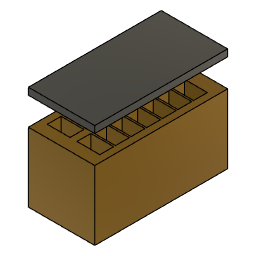
Sertraline 50or100 v0 (Autodesk Fusion 360 design; units mm, degrees)
Autodesk Fusion 360 part; units mm, degrees
note: some values were not read from the file. Chosen so that the rebuilt part matches the saved one: which face or edge a step refers to; a direction.
sketch "Sketch1" plane through (0, 0, 0) normal (0, 0, 1) x (1, 0, 0)
  line L0 (32.9923, 14.7897) -> (80.9923, 14.7897)
  line L1 (80.9923, 14.7897) -> (80.9923, 110.7897)
  line L2 (80.9923, 110.7897) -> (32.9923, 110.7897)
  line L3 (32.9923, 110.7897) -> (32.9923, 14.7897)
  line L4 (56.9923, 110.7897) -> (56.9923, 14.7897)
  line L5 (56.9923, 110.7897) -> (56.9923, 101.7897)
  line L6 (56.9923, 14.7897) -> (56.9923, 22.7897)
  line L7 (56.9923, 22.7897) -> (56.9923, 34.0754)
  line L8 (56.9923, 34.0754) -> (56.9923, 45.3611)
  line L9 (56.9923, 45.3611) -> (56.9923, 56.6468)
  line L10 (56.9923, 56.6468) -> (56.9923, 67.9325)
  line L11 (56.9923, 67.9325) -> (56.9923, 79.2182)
  line L12 (56.9923, 79.2182) -> (56.9923, 90.5039)
  line L13 (56.9923, 90.5039) -> (56.9923, 101.7897)
  line L14 (56.9923, 101.7897) -> (56.9923, 101.1468)
  line L15 (56.9923, 90.5039) -> (56.9923, 91.1468)
  line L16 (56.9923, 90.5039) -> (56.9923, 89.8611)
  line L17 (56.9923, 79.2182) -> (56.9923, 79.8611)
  line L18 (56.9923, 79.2182) -> (56.9923, 78.5754)
  line L19 (56.9923, 67.9325) -> (56.9923, 68.5754)
  line L20 (56.9923, 67.9325) -> (56.9923, 67.2897)
  line L21 (56.9923, 56.6468) -> (56.9923, 57.2897)
  line L22 (56.9923, 56.6468) -> (56.9923, 56.0039)
  line L23 (56.9923, 45.3611) -> (56.9923, 46.0039)
  line L24 (56.9923, 45.3611) -> (56.9923, 44.7182)
  line L25 (56.9923, 34.0754) -> (56.9923, 34.7182)
  line L26 (56.9923, 34.0754) -> (56.9923, 33.4325)
  line L27 (56.9923, 22.7897) -> (56.9923, 23.4325)
  line L28 (32.9923, 101.1468) -> (80.9923, 101.1468)
  line L29 (80.9923, 91.1468) -> (32.9923, 91.1468)
  line L30 (80.9923, 89.8611) -> (32.9923, 89.8611)
  line L31 (80.9923, 79.8611) -> (32.9923, 79.8611)
  line L32 (80.9923, 78.5754) -> (32.9923, 78.5754)
  line L33 (80.9923, 68.5754) -> (32.9923, 68.5754)
  line L34 (80.9923, 67.2897) -> (32.9923, 67.2897)
  line L35 (80.9923, 57.2897) -> (32.9923, 57.2897)
  line L36 (80.9923, 56.0039) -> (32.9923, 56.0039)
  line L37 (80.9923, 46.0039) -> (32.9923, 46.0039)
  line L38 (80.9923, 44.7182) -> (32.9923, 44.7182)
  line L39 (80.9923, 34.7182) -> (32.9923, 34.7182)
  line L40 (80.9923, 33.4325) -> (32.9923, 33.4325)
  line L41 (80.9923, 23.4325) -> (32.9923, 23.4325)
  dimension "d1" = 48
  dimension "d2" = 96
  dimension "d3" = 9
  dimension "d4" = 8
  dimension "d5" = 11.2857
  dimension "d6" = 11.2857
  dimension "d7" = 11.2857
  dimension "d8" = 11.2857
  dimension "d9" = 11.2857
  dimension "d10" = 11.2857
  dimension "d11" = 11.2857
  dimension "d13" = 0.6429
  dimension "d14" = 0.6429
  dimension "d15" = 0.6429
  dimension "d16" = 0.6429
  dimension "d17" = 0.6429
  dimension "d18" = 0.6429
  dimension "d19" = 0.6429
  dimension "d20" = 0.6429
  dimension "d21" = 0.6429
  dimension "d22" = 0.6429
  dimension "d23" = 0.6429
  dimension "d24" = 0.6429
  dimension "d25" = 0.6429
  dimension "d26" = 0.6429
  constraint horizontal L0
  constraint vertical L1
  constraint horizontal L2
  constraint vertical L3
  constraint midpoint L2 L4.start
  constraint midpoint L0 L4.end
  constraint perpendicular L2 L5
  constraint perpendicular L0 L6
  constraint parallel L4 L7
  constraint parallel L4 L8
  constraint parallel L4 L9
  constraint parallel L4 L10
  constraint coincident L4 L11.end
  constraint coincident L4 L12.end
  constraint parallel L4 L13
  constraint vertical L14
  constraint vertical L15
  constraint parallel L4 L16
  constraint vertical L17
  constraint vertical L18
  constraint vertical L19
  constraint vertical L20
  constraint vertical L21
  constraint vertical L22
  constraint vertical L23
  constraint parallel L4 L24
  constraint parallel L8 L25
  constraint parallel L4 L26
  constraint parallel L4 L27
  constraint coincident L3 L28.start
  constraint coincident L1 L28.end
  constraint perpendicular L1 L28
  constraint coincident L1 L29.start
  constraint coincident L3 L29.end
  constraint perpendicular L3 L29
  constraint coincident L1 L30.start
  constraint coincident L3 L30.end
  constraint perpendicular L3 L30
  constraint coincident L1 L31.start
  constraint coincident L3 L31.end
  constraint perpendicular L3 L31
  constraint coincident L1 L32.start
  constraint coincident L3 L32.end
  constraint perpendicular L3 L32
  constraint coincident L1 L33.start
  constraint coincident L3 L33.end
  constraint perpendicular L3 L33
  constraint coincident L1 L34.start
  constraint coincident L3 L34.end
  constraint perpendicular L3 L34
  constraint coincident L3 L35.end
  constraint perpendicular L3 L35
  constraint coincident L1 L36.start
  constraint coincident L3 L36.end
  constraint perpendicular L3 L36
  constraint coincident L1 L37.start
  constraint coincident L3 L37.end
  constraint perpendicular L3 L37
  constraint coincident L3 L38.end
  constraint perpendicular L3 L38
  constraint coincident L1 L39.start
  constraint coincident L3 L39.end
  constraint perpendicular L3 L39
  constraint coincident L1 L40.start
  constraint coincident L3 L40.end
  constraint perpendicular L3 L40
  constraint coincident L1 L41.start
  constraint coincident L3 L41.end
  constraint perpendicular L3 L41
  measures "d1" distance of L0.start L0.end
  measures "d2" distance of L0.start L2.end
  measures "d3" distance of L4.start L5.end
  measures "d4" distance of L4.end L6.end
  measures "d5" distance of L6.end L7.end
  measures "d6" distance of L7.end L8.end
  measures "d7" distance of L8.end L9.end
  measures "d8" distance of L9.end L10.end
  measures "d9" distance of L10.end L11.end
  measures "d10" distance of L11.end L12.end
  measures "d11" distance of L12.end L5.end
  measures "d13" distance of L5.end L14.end
  measures "d14" distance of L12.end L15.end
  measures "d15" distance of L12.end L16.end
  measures "d16" distance of L11.end L17.end
  measures "d17" distance of L11.end L18.end
  measures "d18" distance of L10.end L19.end
  measures "d19" distance of L10.end L20.end
  measures "d20" distance of L9.end L21.end
  measures "d21" distance of L9.end L22.end
  measures "d22" distance of L8.end L23.end
  measures "d23" distance of L8.end L24.end
  measures "d24" distance of L7.end L25.end
  measures "d25" distance of L7.end L26.end
  measures "d26" distance of L6.end L27.end
extrude "Extrude1" add sketch "Sketch1" along normal blind 5 contours L0 L3 L4 L6 L7 L27 L41 | L0 L1 L4 L6 L7 L27 L41 | L3 L4 L7 L40 L41 | L1 L4 L7 L40 L41 | L3 L4 L8 L38 L39 | L1 L4 L8 L38 L39 | L3 L4 L9 L36 L37 | L1 L4 L9 L36 L37 | L3 L4 L10 L34 L35 | L1 L4 L10 L34 L35 | L3 L4 L11 L32 L33 | L1 L4 L11 L32 L33 | L3 L4 L12 L30 L31 | L1 L4 L12 L30 L31 | L3 L4 L13 L28 L29 | L2 L3 L4 L5 L13 L14 L28 | L1 L4 L13 L28 L29 | L1 L2 L4 L5 L13 L14 L28 makes body 1 at (48.9923, 49.3373, 0) makes body 2 at (64.9923, 97.6944, 0) makes body 3 at (48.9923, 60.623, 0) makes body 4 at (48.9923, 38.0516, 0) makes body 5 at (48.9923, 83.1944, 0) makes body 6 at (48.9923, 71.9087, 0) makes body 7 at (64.9923, 21.0039, 0)
sketch "Sketch2" plane through (0, 0, 5) normal (0, 0, 1) x (-1, 0, 0)
  line L0 (-80.9923, -110.7897) -> (-32.9923, -110.7897)
  line L1 (-32.9923, -110.7897) -> (-32.9923, -91.1468)
  line L2 (-32.9923, -91.1468) -> (-80.9923, -91.1468)
  line L3 (-80.9923, -91.1468) -> (-80.9923, -110.7897)
  line L4 (-32.9923, -110.7897) -> (-80.9923, -110.7897)
  line L5 (-80.9923, -110.7897) -> (-80.9923, -14.7897)
  line L6 (-80.9923, -14.7897) -> (-32.9923, -14.7897)
  line L7 (-32.9923, -14.7897) -> (-32.9923, -110.7897)
  point P0 (-80.9923, -14.7897)
  constraint horizontal L4
  constraint vertical L5
  constraint horizontal L6
  constraint vertical L7
  constraint coincident P0 L5.end
  constraint coincident L0.end L1.start
extrude "Extrude2" add sketch "Sketch2" along normal blind 5 bodies 1 2 3 4 5 6 7
sketch "Sketch3" plane through (0, 0, 0) normal (0, 0, -1) x (1, 0, 0)
  line L0 (32.9923, -67.2897) -> (80.9923, -67.2897)
  line L1 (80.9923, -67.2897) -> (80.9923, -57.2897)
  line L2 (80.9923, -57.2897) -> (32.9923, -57.2897)
  line L3 (32.9923, -57.2897) -> (32.9923, -67.2897)
  line L4 (56.9923, -62.2897) -> (56.9923, -10.4261)
  line L5 (56.9923, -10.4261) -> (54.4923, -10.4261)
  line L6 (54.4923, -10.4261) -> (59.4923, -10.4261)
  line L7 (59.4923, -10.4261) -> (59.4923, -116.1446)
  line L8 (59.4923, -116.1446) -> (54.4923, -116.1446)
  line L9 (54.4923, -116.1446) -> (54.4923, -10.4261)
  dimension "d32" = 2.5
  dimension "d33" = 5
  constraint perpendicular L2 L4
  constraint perpendicular L4 L5
  constraint horizontal L6
  constraint vertical L7
  constraint horizontal L8
  constraint vertical L9
  measures "d32" distance of L4.end L5.end
  measures "d33" distance of L5.end L6.end
extrude "Extrude3" cut sketch "Sketch3" against normal blind 5 contours L0 L2 L7 L9 | L0 L7 L8 L9 | L2 L4 L5 L6 L9 | L2 L4 L6 L7 bodies 1
sketch "Sketch4" plane through (0, 0, 0) normal (0, 0, 1) x (1, 0, 0)
extrude "Extrude4" cut sketch "Sketch1" along normal blind 5 contours L2 L3 L4 L5 L13 L14 L28 | L1 L2 L4 L5 L13 L14 L28 bodies 1
extrude "Extrude5" cut sketch "Sketch1" along normal blind 5 contours L0 L3 L4 L6 L7 L27 L41 | L0 L1 L4 L6 L7 L27 L41 bodies 1
sketch "Sketch5" plane through (0, 0, 0) normal (0, 0, 1) x (1, 0, 0)
  line L0 (80.9923, 14.7897) -> (75.9923, 14.7897)
  line L1 (32.9923, 14.7897) -> (37.9923, 14.7897)
  line L2 (32.9923, 14.7897) -> (37.9923, 14.7897)
  line L3 (37.9923, 14.7897) -> (37.9923, 110.7897)
  line L4 (37.9923, 110.7897) -> (32.9923, 110.7897)
  line L5 (32.9923, 110.7897) -> (32.9923, 14.7897)
  line L6 (80.9923, 110.7897) -> (32.9923, 110.7897)
  line L7 (75.9923, 14.7897) -> (80.9923, 14.7897)
  line L8 (80.9923, 14.7897) -> (80.9923, 110.7897)
  line L9 (80.9923, 110.7897) -> (75.9923, 110.7897)
  line L10 (75.9923, 110.7897) -> (75.9923, 14.7897)
  point P0 (80.9923, 14.7897)
  point P1 (32.9923, 14.7897)
  dimension "d40" = 5
  dimension "d41" = 5
  constraint coincident P0 L0.start
  constraint coincident P1 L1.start
  constraint horizontal L2
  constraint vertical L3
  constraint horizontal L4
  constraint vertical L5
  constraint coincident L3.end L6
  constraint horizontal L7
  constraint vertical L8
  constraint horizontal L9
  constraint vertical L10
  constraint coincident L6.start L8.end
  measures "d40" distance of P0 L0.end
  measures "d41" distance of P1 L1.end
extrude "Extrude6" cut sketch "Sketch5" along normal blind 5 bodies 1
extrude "Extrude7" add sketch "Sketch3" sketch "Sketch5" sketch "Sketch1" against normal blind 25 separate body contours L0 L2 L7 L9 | L0 L7 L8 L9 | L2 L4 L5 L6 L9 | L2 L4 L6 L7 of sketch 2 of sketch 3 contours L0 L3 L4 L6 L7 L27 L41 | L0 L1 L4 L6 L7 L27 L41 | L3 L4 L7 L8 L25 L26 L39 L40 | L1 L4 L7 L8 L25 L26 L39 L40 | L3 L4 L8 L9 L23 L24 L37 L38 | L1 L4 L8 L9 L23 L24 L37 L38 | L3 L4 L9 L10 L21 L22 L35 L36 | L1 L4 L9 L10 L21 L22 L35 L36 | L3 L4 L10 L11 L19 L20 L33 L34 | L1 L4 L10 L11 L19 L20 L33 L34 | L3 L4 L11 L12 L17 L18 L31 L32 | L1 L4 L11 L12 L17 L18 L31 L32 | L3 L4 L12 L13 L15 L16 L29 L30 | L1 L4 L12 L13 L15 L16 L29 L30 | L2 L3 L4 L5 L13 L14 L28 | L1 L2 L4 L5 L13 L14 L28 makes body 8
move_body "Move1" bodies 8 to x (1, 0, 0) y (0, 1, 0) z (0, 0, 1) at (0, 0, -40)
split "Split1" by plane through (56.9923, 110.7897, -40) normal (0, 1, 0) and through (32.9923, 14.7897, -40) normal (0, -1, 0) bodies 8 makes body 9 at (59.4923, 112.5746, -31.6667) makes body 10 at (57.8256, 10.4261, -31.6667)
delete_body "RemoveBody1" bodies 9
delete_body "RemoveBody2" bodies 10
extrude "Extrude8" cut 1 faces at (72.159, 107.5754, -40) along direction (0, 0, 1) blind 10 on bodies 8 bodies 8
sketch "Sketch6" plane through (0, 0, -30) normal (0, 0, -1) x (1, 0, 0)
  line L0 (37.9923, -91.1468) -> (54.4923, -91.1468)
  line L1 (54.4923, -91.1468) -> (54.4923, -101.1468)
  line L2 (54.4923, -101.1468) -> (37.9923, -101.1468)
  line L3 (37.9923, -101.1468) -> (37.9923, -91.1468)
  line L4 (75.9923, -68.5754) -> (75.9923, -78.5754)
  line L5 (75.9923, -78.5754) -> (59.4923, -78.5754)
  line L6 (59.4923, -78.5754) -> (59.4923, -68.5754)
  line L7 (59.4923, -68.5754) -> (75.9923, -68.5754)
  line L8 (37.9923, -67.2897) -> (37.9923, -57.2897)
  line L9 (37.9923, -57.2897) -> (54.4923, -57.2897)
  line L10 (54.4923, -57.2897) -> (54.4923, -67.2897)
  line L11 (54.4923, -67.2897) -> (37.9923, -67.2897)
  line L12 (75.9923, -67.2897) -> (59.4923, -67.2897)
  line L13 (59.4923, -67.2897) -> (59.4923, -57.2897)
  line L14 (59.4923, -57.2897) -> (75.9923, -57.2897)
  line L15 (75.9923, -57.2897) -> (75.9923, -67.2897)
  line L16 (37.9923, -46.0039) -> (54.4923, -46.0039)
  line L17 (54.4923, -46.0039) -> (54.4923, -56.0039)
  line L18 (54.4923, -56.0039) -> (37.9923, -56.0039)
  line L19 (37.9923, -56.0039) -> (37.9923, -46.0039)
  line L20 (37.9923, -23.4325) -> (54.4923, -23.4325)
  line L21 (54.4923, -23.4325) -> (54.4923, -33.4325)
  line L22 (54.4923, -33.4325) -> (37.9923, -33.4325)
  line L23 (37.9923, -33.4325) -> (37.9923, -23.4325)
  line L24 (75.9923, -23.4325) -> (75.9923, -33.4325)
  line L25 (75.9923, -33.4325) -> (59.4923, -33.4325)
  line L26 (59.4923, -33.4325) -> (59.4923, -23.4325)
  line L27 (59.4923, -23.4325) -> (75.9923, -23.4325)
  line L28 (75.9923, -44.7182) -> (59.4923, -44.7182)
  line L29 (59.4923, -44.7182) -> (59.4923, -34.7182)
  line L30 (59.4923, -34.7182) -> (75.9923, -34.7182)
  line L31 (75.9923, -34.7182) -> (75.9923, -44.7182)
  line L32 (37.9923, -44.7182) -> (37.9923, -34.7182)
  line L33 (37.9923, -34.7182) -> (54.4923, -34.7182)
  line L34 (54.4923, -34.7182) -> (54.4923, -44.7182)
  line L35 (54.4923, -44.7182) -> (37.9923, -44.7182)
  line L36 (75.9923, -46.0039) -> (75.9923, -56.0039)
  line L37 (75.9923, -56.0039) -> (59.4923, -56.0039)
  line L38 (59.4923, -56.0039) -> (59.4923, -46.0039)
  line L39 (59.4923, -46.0039) -> (75.9923, -46.0039)
  line L40 (37.9923, -68.5754) -> (54.4923, -68.5754)
  line L41 (54.4923, -68.5754) -> (54.4923, -78.5754)
  line L42 (54.4923, -78.5754) -> (37.9923, -78.5754)
  line L43 (37.9923, -78.5754) -> (37.9923, -68.5754)
  line L44 (75.9923, -89.8611) -> (59.4923, -89.8611)
  line L45 (59.4923, -89.8611) -> (59.4923, -79.8611)
  line L46 (59.4923, -79.8611) -> (75.9923, -79.8611)
  line L47 (75.9923, -79.8611) -> (75.9923, -89.8611)
  line L48 (37.9923, -89.8611) -> (37.9923, -79.8611)
  line L49 (37.9923, -79.8611) -> (54.4923, -79.8611)
  line L50 (54.4923, -79.8611) -> (54.4923, -89.8611)
  line L51 (54.4923, -89.8611) -> (37.9923, -89.8611)
  line L52 (75.9923, -91.1468) -> (75.9923, -101.1468)
  line L53 (75.9923, -101.1468) -> (59.4923, -101.1468)
  line L54 (59.4923, -101.1468) -> (59.4923, -91.1468)
  line L55 (59.4923, -91.1468) -> (75.9923, -91.1468)
  line L56 (80.9923, -14.7897) -> (32.9923, -14.7897)
  line L57 (32.9923, -14.7897) -> (32.9923, -110.7897)
  line L58 (32.9923, -110.7897) -> (80.9923, -110.7897)
  line L59 (80.9923, -110.7897) -> (80.9923, -14.7897)
  line L60 (37.9923, -101.1468) -> (75.9923, -101.1468)
  line L61 (75.9923, -101.1468) -> (75.9923, -110.7897)
  line L62 (75.9923, -110.7897) -> (37.9923, -110.7897)
  line L63 (37.9923, -110.7897) -> (37.9923, -101.1468)
  line L64 (37.9923, -101.1468) -> (75.9923, -101.1468)
  line L65 (75.9923, -101.1468) -> (75.9923, -23.4325)
  line L66 (75.9923, -23.4325) -> (37.9923, -23.4325)
  line L67 (37.9923, -23.4325) -> (37.9923, -101.1468)
  constraint horizontal L60
  constraint vertical L61
  constraint horizontal L62
  constraint vertical L63
  constraint coincident L58 L61.end
  constraint coincident L2.end L3.start
  constraint horizontal L64
  constraint vertical L65
  constraint horizontal L66
  constraint vertical L67
  constraint coincident L24.start L27.end
extrude "Extrude9" add sketch "Sketch6" along normal blind 30 contours L3 L4 L8 L15 L19 L20 L23 L24 L27 L31 L32 L36 L43 L47 L48 L52 L56 L57 L58 L59 L61 L63 L65 L66 L67 bodies 8
sketch "Sketch7" plane through (0, 0, -60) normal (0, 0, -1) x (1, 0, 0)
  line L0 (75.9923, -23.4325) -> (75.9923, -110.7897)
  line L1 (75.9923, -110.7897) -> (80.9923, -110.7897)
  line L2 (80.9923, -110.7897) -> (80.9923, -14.7897)
  line L3 (80.9923, -14.7897) -> (32.9923, -14.7897)
  line L4 (32.9923, -14.7897) -> (32.9923, -110.7897)
  line L5 (32.9923, -110.7897) -> (37.9923, -110.7897)
  line L6 (37.9923, -110.7897) -> (37.9923, -23.4325)
  line L7 (37.9923, -23.4325) -> (75.9923, -23.4325)
  line L8 (32.9923, -14.7897) -> (80.9923, -14.7897)
  line L9 (80.9923, -14.7897) -> (80.9923, -110.7897)
  line L10 (80.9923, -110.7897) -> (32.9923, -110.7897)
  line L11 (32.9923, -110.7897) -> (32.9923, -14.7897)
  constraint horizontal L8
  constraint vertical L9
  constraint horizontal L10
  constraint vertical L11
  constraint coincident L1.end L2.start
  constraint coincident L3.end L4.start
extrude "Extrude10" add sketch "Sketch7" along normal blind 5 bodies 8
sketch "Sketch8" plane through (0, 0, -30) normal (0, 0, -1) x (1, 0, 0)
  line L0 (37.9923, -101.1468) -> (37.9923, -110.7897)
  line L1 (37.9923, -110.7897) -> (75.9923, -110.7897)
  line L2 (75.9923, -110.7897) -> (75.9923, -101.1468)
  line L3 (75.9923, -101.1468) -> (59.4923, -101.1468)
  line L4 (59.4923, -101.1468) -> (59.4923, -91.1468)
  line L5 (59.4923, -91.1468) -> (75.9923, -91.1468)
  line L6 (75.9923, -91.1468) -> (75.9923, -89.8611)
  line L7 (75.9923, -89.8611) -> (59.4923, -89.8611)
  line L8 (59.4923, -89.8611) -> (59.4923, -79.8611)
  line L9 (59.4923, -79.8611) -> (75.9923, -79.8611)
  line L10 (75.9923, -79.8611) -> (75.9923, -78.5754)
  line L11 (75.9923, -78.5754) -> (59.4923, -78.5754)
  line L12 (59.4923, -78.5754) -> (59.4923, -68.5754)
  line L13 (59.4923, -68.5754) -> (75.9923, -68.5754)
  line L14 (75.9923, -68.5754) -> (75.9923, -67.2897)
  line L15 (75.9923, -67.2897) -> (59.4923, -67.2897)
  line L16 (59.4923, -67.2897) -> (59.4923, -57.2897)
  line L17 (59.4923, -57.2897) -> (75.9923, -57.2897)
  line L18 (75.9923, -57.2897) -> (75.9923, -56.0039)
  line L19 (75.9923, -56.0039) -> (59.4923, -56.0039)
  line L20 (59.4923, -56.0039) -> (59.4923, -46.0039)
  line L21 (59.4923, -46.0039) -> (75.9923, -46.0039)
  line L22 (75.9923, -46.0039) -> (75.9923, -44.7182)
  line L23 (75.9923, -44.7182) -> (59.4923, -44.7182)
  line L24 (59.4923, -44.7182) -> (59.4923, -34.7182)
  line L25 (59.4923, -34.7182) -> (75.9923, -34.7182)
  line L26 (75.9923, -34.7182) -> (75.9923, -33.4325)
  line L27 (75.9923, -33.4325) -> (59.4923, -33.4325)
  line L28 (59.4923, -33.4325) -> (59.4923, -23.4325)
  line L29 (59.4923, -23.4325) -> (54.4923, -23.4325)
  line L30 (54.4923, -23.4325) -> (54.4923, -33.4325)
  line L31 (54.4923, -33.4325) -> (37.9923, -33.4325)
  line L32 (37.9923, -33.4325) -> (37.9923, -34.7182)
  line L33 (37.9923, -34.7182) -> (54.4923, -34.7182)
  line L34 (54.4923, -34.7182) -> (54.4923, -44.7182)
  line L35 (54.4923, -44.7182) -> (37.9923, -44.7182)
  line L36 (37.9923, -44.7182) -> (37.9923, -46.0039)
  line L37 (37.9923, -46.0039) -> (54.4923, -46.0039)
  line L38 (54.4923, -46.0039) -> (54.4923, -56.0039)
  line L39 (54.4923, -56.0039) -> (37.9923, -56.0039)
  line L40 (37.9923, -56.0039) -> (37.9923, -57.2897)
  line L41 (37.9923, -57.2897) -> (54.4923, -57.2897)
  line L42 (54.4923, -57.2897) -> (54.4923, -67.2897)
  line L43 (54.4923, -67.2897) -> (37.9923, -67.2897)
  line L44 (37.9923, -67.2897) -> (37.9923, -68.5754)
  line L45 (37.9923, -68.5754) -> (54.4923, -68.5754)
  line L46 (54.4923, -68.5754) -> (54.4923, -78.5754)
  line L47 (54.4923, -78.5754) -> (37.9923, -78.5754)
  line L48 (37.9923, -78.5754) -> (37.9923, -79.8611)
  line L49 (37.9923, -79.8611) -> (54.4923, -79.8611)
  line L50 (54.4923, -79.8611) -> (54.4923, -89.8611)
  line L51 (54.4923, -89.8611) -> (37.9923, -89.8611)
  line L52 (37.9923, -89.8611) -> (37.9923, -91.1468)
  line L53 (37.9923, -91.1468) -> (54.4923, -91.1468)
  line L54 (54.4923, -91.1468) -> (54.4923, -101.1468)
  line L55 (54.4923, -101.1468) -> (37.9923, -101.1468)
  line L56 (75.9923, -101.1468) -> (37.9923, -101.1468)
  line L57 (37.9923, -101.1468) -> (37.9923, -110.7897)
  line L58 (37.9923, -110.7897) -> (75.9923, -110.7897)
  line L59 (75.9923, -110.7897) -> (75.9923, -101.1468)
  constraint horizontal L56
  constraint vertical L57
  constraint horizontal L58
  constraint vertical L59
  constraint coincident L0.end L1.start
  constraint coincident L2.end L3.start
extrude "Extrude11" add sketch "Sketch8" along normal blind 20 contours L0 L1 L2 L3 L55 L56 L57 L58 L59 bodies 8
move_face "OffsetFaces1" offset -0.5 7 faces at (75.9923, 41.3849, 1.6667) (75.9923, 30.0992, 1.6667) (75.9923, 52.6706, 1.6667) (75.9923, 63.9563, 1.6667) (75.9923, 75.242, 1.6667) (75.9923, 86.5277, 1.6667) (75.9923, 97.8135, 1.6667) on bodies 1
extrude "Extrude12" cut 7 faces at (37.9923, 97.8135, 3.3333) (37.9923, 86.5277, 3.3333) (37.9923, 75.242, 3.3333) (37.9923, 63.9563, 3.3333) (37.9923, 52.6706, 3.3333) (37.9923, 41.3849, 3.3333) (37.9923, 30.0992, 3.3333) along direction (1, 0, 0) blind 0.5 on bodies 1 bodies 1
extrude "Extrude13" cut 2 faces at (64.8256, 91.1468, 3.3333) (43.8256, 91.1468, 3.3333) along direction (0, 1, 0) blind 0.5 on bodies 1 bodies 1
extrude "Extrude14" cut 2 faces at (43.8256, 79.8611, 3.3333) (64.8256, 79.8611, 3.3333) along direction (0, 1, 0) blind 0.5 on bodies 1 bodies 1
extrude "Extrude15" cut 2 faces at (43.8256, 68.5754, 3.3333) (64.8256, 68.5754, 3.3333) along direction (0, 1, 0) blind 0.5 on bodies 1 bodies 1
extrude "Extrude16" cut 2 faces at (43.8256, 57.2897, 3.3333) (64.8256, 57.2897, 3.3333) along direction (0, 1, 0) blind 0.5 on bodies 1 bodies 1
extrude "Extrude17" cut 2 faces at (43.8256, 46.0039, 3.3333) (64.8256, 46.0039, 3.3333) along direction (0, 1, 0) blind 0.5 on bodies 1 bodies 1
extrude "Extrude18" cut 2 faces at (64.8256, 34.7182, 3.3333) (43.8256, 34.7182, 3.3333) along direction (0, 1, 0) blind 0.5 on bodies 1 bodies 1
extrude "Extrude19" cut 2 faces at (64.8256, 23.4325, 3.3333) (43.8256, 23.4325, 3.3333) along direction (0, 1, 0) blind 0.5 on bodies 1 bodies 1
extrude "Extrude20" cut 7 faces at (59.4923, 30.2658, 3.3333) (59.4923, 41.5516, 3.3333) (59.4923, 52.8373, 3.3333) (59.4923, 64.123, 3.3333) (59.4923, 72.242, 3.3333) (59.4923, 86.6944, 3.3333) (59.4923, 97.9801, 3.3333) along direction (1, 0, 0) blind 0.5 on bodies 1 bodies 1
extrude "Extrude21" cut 7 faces at (54.4923, 27.0992, 3.3333) (54.4923, 41.5516, 3.3333) (54.4923, 49.6706, 3.3333) (54.4923, 60.9563, 3.3333) (54.4923, 72.242, 3.3333) (54.4923, 83.5277, 3.3333) (54.4923, 97.9801, 3.3333) along direction (-1, 0, 0) blind 0.5 on bodies 1 bodies 1
extrude "Extrude22" cut 2 faces at (43.659, 101.1468, 3.3333) (65.159, 101.1468, 3.3333) along direction (0, -1, 0) blind 0.5 on bodies 1 bodies 1
extrude "Extrude23" cut 2 faces at (48.8256, 89.8611, 3.3333) (65.159, 89.8611, 3.3333) along direction (0, -1, 0) blind 0.5 on bodies 1 bodies 1
extrude "Extrude24" cut 2 faces at (48.8256, 78.5754, 3.3333) (65.159, 78.5754, 3.3333) along direction (0, -1, 0) blind 0.5 on bodies 1 bodies 1
extrude "Extrude25" cut 2 faces at (48.8256, 67.2897, 3.3333) (65.159, 67.2897, 3.3333) along direction (0, -1, 0) blind 0.5 on bodies 1 bodies 1
extrude "Extrude26" cut 2 faces at (48.8256, 56.0039, 3.3333) (65.159, 56.0039, 3.3333) along direction (0, -1, 0) blind 0.5 on bodies 1 bodies 1
extrude "Extrude27" cut 2 faces at (48.8256, 44.7182, 3.3333) (65.159, 44.7182, 3.3333) along direction (0, -1, 0) blind 0.5 on bodies 1 bodies 1
extrude "Extrude28" cut 2 faces at (65.159, 33.4325, 3.3333) (48.8256, 33.4325, 3.3333) along direction (0, -1, 0) blind 0.5 on bodies 1 bodies 1
equation "d13 = ( 1.2857143 / 2 ) * 1 mm"
equation "d14 = ( 1.2857143 / 2 ) * 1 mm"
equation "d15 = ( 1.2857143 / 2 ) * 1 mm"
equation "d16 = ( 1.2857143 / 2 ) * 1 mm"
equation "d17 = ( 1.2857143 / 2 ) * 1 mm"
equation "d18 = ( 1.2857143 / 2 ) * 1 mm"
equation "d19 = ( 1.2857143 / 2 ) * 1 mm"
equation "d20 = ( 1.2857143 / 2 ) * 1 mm"
equation "d21 = ( 1.2857143 / 2 ) * 1 mm"
equation "d22 = ( 1.2857143 / 2 ) * 1 mm"
equation "d23 = ( 1.2857143 / 2 ) * 1 mm"
equation "d24 = ( 1.2857143 / 2 ) * 1 mm"
equation "d25 = ( 1.2857143 / 2 ) * 1 mm"
equation "d26 = ( 1.2857143 / 2 ) * 1 mm"
equation "d44 = 5 mm - 30 mm"
